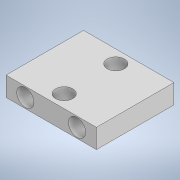
# Autodesk Inventor part: XL_XL_interface_v2
Saved by Autodesk Inventor 2021 (Build 250183000, 183)
## iProperties
Created: 2020-11-17
Part Number: XL_XL_interface_v2
Material: Generic
Document SubType Name: Modeling
Designer: Paco
Density: 1 g/cm^3
Appearance: Default
Mass: 1.13551 g
Surface Area: 15.7196 cm^2
Volume: 1.13551 cm^3
Author: Paco
Autodesk Inventor part; units mm, degrees
ref_plane "YZ Plane" through (0, 0, 0) normal (1, 0, 0) x (0, 1, 0)
ref_plane "XZ Plane" through (0, 0, 0) normal (0, 1, 0) x (-1, 0, 0)
ref_plane "XY Plane" through (0, 0, 0) normal (0, 0, 1) x (1, 0, 0)
sketch "Sketch1" plane through (0, 0, 0) normal (1, 0, 0) x (0, 1, 0)
  line L0 (3.2881, 15.1027) -> (-1.2119, 15.1027)
  line L1 (-1.2119, 15.1027) -> (-1.2119, -2.8973)
  line L2 (-1.2119, -2.8973) -> (3.2881, -2.8973)
  line L3 (3.2881, -2.8973) -> (3.2881, 15.1027)
  point P0 (0, 0)
  dimension "d0" = 4.5
  dimension "d1" = 18
  constraints: 8 end point, 2 parallel, 1 horizontal, 1 perpendicular
  measures "d0" distance of L1.end L2.end
  measures "d1" distance of L0.end L1.end
extrude "Extrusion1" add sketch "Sketch1" along normal blind 21
sketch "Sketch2" plane through (0, 3.2881, 15.1027) normal (0, 1, 0) x (1, 0, 0)
  circle A0 centre (10.5, 3) radius 2
  circle A1 centre (10.5, 3) radius 2
  circle A2 centre (10.5, 15) radius 2
  line L0 (0, 18) -> (21, 18) projected
  line L1 (0, 0) -> (21, 0) projected
  line L2 (0, 18) -> (0, 0) projected
  point P0 (0, 15.1027)
  dimension "d4" = 18
  dimension "d5" = 12
  dimension "d6" = 3
  dimension "d7" = 10.5
  dimension "d8" = 21
  dimension "d9" = 10.5
  constraints: 3 centre point, 1 coincident
  measures "d4" distance between parallel lines of L0 L1
  measures "d5" distance of A2.centre A1.centre
  measures "d6" distance from line of L1 A1.centre
  measures "d7" distance from line of L2 A1.centre
  measures "d8" distance of L0.start L0.end
  measures "d9" distance from line of L2 A2.centre
sketch "Sketch3" plane through (0, -1.2119, -2.8973) normal (0, 0, -1) x (-1, 0, 0)
  circle A0 centre (-4.5, 2.25) radius 2
  circle A1 centre (-4.5, 2.25) radius 2
  circle A2 centre (-16.5, 2.25) radius 2
  line L0 (0, 4.5) -> (-21, 4.5) projected
  line L1 (0, 0) -> (0, 4.5) projected
  point P0 (0, 1.2119)
  dimension "d10" = 12
  dimension "d11" = 2.25
  dimension "d12" = 2.25
  dimension "d13" = 4.5
  constraints: 3 centre point, 1 coincident
  measures "d10" distance of A2.centre A1.centre
  measures "d11" distance from line of L0 A1.centre
  measures "d12" distance from line of L0 A2.centre
  measures "d13" distance from line of L1 A1.centre
extrude "Extrusion2" cut sketch "Sketch2" against normal through all
extrude "Extrusion3" cut sketch "Sketch3" against normal through all
equation "\"d7\" = 0.5 * d8"
equation "\"d9\" = d7"
equation "\"d12\" = d11"
body "Solid1"
